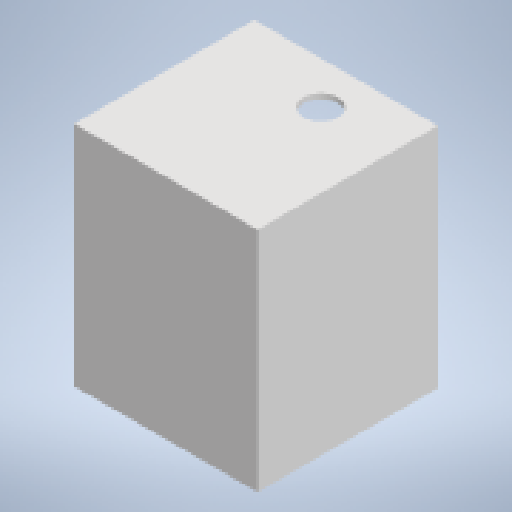
# Autodesk Inventor part: HANG
Saved by Autodesk Inventor 2023.2 (Build 272271030, 271C)
## iProperties
Created: 2023-06-22
Part Number: HANG
Material: Generic
Document SubType Name: Modeling
Designer: kao91
Density: 1 g/cm^3
Appearance: Default
Author: kao91
Autodesk Inventor part; units mm, degrees
ref_plane "YZ Plane" through (0, 0, 0) normal (1, 0, 0) x (0, 1, 0)
ref_plane "XZ Plane" through (0, 0, 0) normal (0, 1, 0) x (-1, 0, 0)
ref_plane "XY Plane" through (0, 0, 0) normal (0, 0, 1) x (1, 0, 0)
sketch "Sketch1" plane through (0, 0, 0) normal (0, 0, 1) x (1, 0, 0)
  line L0 (52.4625, 25) -> (-52.4625, 25)
  line L1 (-52.4625, 25) -> (-52.4625, -105)
  line L2 (52.4625, -105) -> (52.4625, 25)
  line L3 (-96.7125, -125) -> (96.7125, -125) projected
  line L4 (55.4625, -110) -> (55.4625, -50) projected
  line L5 (-55.4625, -50) -> (-55.4625, -110) projected
  line L6 (52.4625, -105) -> (49.4625, -105)
  line L7 (49.4625, -105) -> (49.4625, 22)
  line L8 (49.4625, 25) -> (52.4625, 25)
  line L9 (52.4625, 25) -> (52.4625, -105)
  line L10 (-52.4625, -105) -> (-49.4625, -105)
  line L11 (-49.4625, -105) -> (-49.4625, 22)
  line L12 (-49.4625, 25) -> (-52.4625, 25)
  line L13 (-52.4625, 25) -> (-52.4625, -105)
  line L14 (49.4625, 25) -> (-49.4625, 25)
  line L15 (-49.4625, 22) -> (49.4625, 22)
  line L16 (-52.4625, -105) -> (-49.4625, -105)
  line L17 (49.4625, -105) -> (52.4625, -105)
  point P0 (0, 0)
  point P1 (50.9625, -105)
  dimension "d7" = 127
  dimension "d8" = 20
  dimension "d9" = 3
  dimension "d10" = 3
  dimension "d11" = 98.925
  dimension "d12" = 3
  dimension "d13" = 3
  constraints: 30 end point, 8 parallel, 4 horizontal, 3 perpendicular, 2 point on line, 1 midpoint
  measures "d7" distance of L6.end L7.end
  measures "d8" distance from line of L3 point (50.963, -105)
  measures "d9" distance between parallel lines of L2 L4
  measures "d10" distance between parallel lines of L5 L13
  measures "d11" distance between parallel lines of L7 L11
  measures "d12" distance between parallel lines of L13 L11
  measures "d13" distance between parallel lines of L15 L0
extrude "Extrusion1" add sketch "Sketch1" along normal blind 100
sketch "Sketch2" plane through (0, 0, 100) normal (0, 0, 1) x (1, 0, 0)
  line L0 (52.4625, -105) -> (52.4625, 25) projected
  line L1 (-52.4625, 25) -> (-52.4625, -105) projected
  line L2 (52.4625, 25) -> (-52.4625, 25)
  line L3 (-52.4625, 25) -> (-52.4625, -105)
  line L4 (-52.4625, -105) -> (52.4625, -105)
  line L5 (52.4625, -105) -> (52.4625, 25)
  point P0 (0, 0)
  constraints: 8 end point, 2 parallel, 1 horizontal, 1 perpendicular
extrude "Extrusion2" add sketch "Sketch2" along normal blind 3
sketch "Sketch3" plane through (-52.4625, -105, 0) normal (-1, 0, 0) x (0, 0, 1)
  circle A0 centre (20, 90) radius 10
  line L0 (0, 130) -> (0, 0) projected
  line L1 (0, 130) -> (103, 130) projected
  point P0 (0, 105)
  dimension "d18" = 20
  dimension "d19" = 20
  dimension "d20" = 40
  constraints: 1 centre point
  measures "d18" diameter of A0
  measures "d19" distance from line of L0 A0.centre
  measures "d20" distance from line of A0.centre L1
extrude "Extrusion3" cut sketch "Sketch3" against normal blind 3
sketch "Sketch4" plane through (-49.4625, 22, 0) normal (0, -1, 0) x (1, 0, 0)
  circle A0 centre (59.3936, 24.3432) radius 10
  point P0 (49.4625, 0)
  dimension "d23" = 20
  constraints: 1 centre point
  measures "d23" diameter of A0
extrude "Extrusion4" cut sketch "Sketch4" against normal blind 3
body "Solid1"
